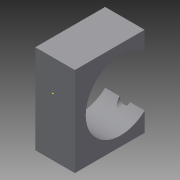
# Autodesk Inventor part: Noke_base
Saved by Autodesk Inventor 2015 SP2 (Build 190223200, 223)
## iProperties
Created: 2016-08-30
Part Number: Noke_base
Material: Generic
Document SubType Name: Modeling
Designer: jm799
Density: 1 g/cm^3
Appearance: Default
Author: jm799
Autodesk Inventor part; units mm, degrees
ref_plane "YZ Plane" through (0, 0, 0) normal (1, 0, 0) x (0, 1, 0)
ref_plane "XZ Plane" through (0, 0, 0) normal (0, 1, 0) x (-1, 0, 0)
ref_plane "XY Plane" through (0, 0, 0) normal (0, 0, 1) x (1, 0, 0)
sketch "Sketch1" plane through (0, 0, 0) normal (0, 1, 0) x (-1, 0, 0)
  line L0 (13.7338, 24.3615) -> (-17.2662, 24.3615)
  line L1 (-17.2662, 24.3615) -> (-17.2662, -45.6385)
  line L2 (-17.2662, -45.6385) -> (13.7338, -45.6385)
  line L3 (13.7338, -45.6385) -> (13.7338, 24.3615)
  point P0 (0, 0)
  dimension "d0" = 31
  dimension "d1" = 70
  constraints: 8 end point, 2 parallel, 1 horizontal, 1 perpendicular
  measures "d0" distance of L0.start L0.end
  measures "d1" distance of L0.end L1.end
extrude "Extrusion1" add sketch "Sketch1" along normal blind 54.75
sketch "Sketch2" plane through (17.2662, 0, 24.3615) normal (1, 0, 0) x (0, 0, -1)
  circle A0 centre (35, 35.9173) radius 27.375
  line L0 (0, 54.75) -> (70, 54.75) construction
  point P0 (24.3615, 0)
  point P1 (35, 54.75)
  dimension "d4" = 54.75
  constraints: 2 end point, 1 centre point, 1 horizontal, 1 midpoint, 1 vertical alignment
  measures "d4" diameter of A0
hole "Hole1" at (17.2662, 35.9173, -10.6385) direction (-1, 0, 0) diameter 54.75 end through all
sketch "Sketch3" plane through (0, 0, 0) normal (0, -1, 0) x (1, 0, 0)
  point P0 (0, 0)
sketch "Sketch4" plane through (0, 54.75, 0) normal (0, 1, 0) x (1, 0, 0)
  line L0 (-13.7338, -9.229) -> (17.2662, -9.229) construction
  line L1 (17.2662, -9.229) -> (-13.7338, -9.229) construction
  circle A0 centre (1.7662, -9.229) radius 4 construction
  point P0 (0, 0)
  dimension "d12" = 8
  constraints: 2 end point, 1 centre point, 1 horizontal, 1 midpoint
  measures "d12" diameter of A0
sketch "Sketch5" plane through (0, 54.75, 0) normal (0, 1, 0) x (1, 0, 0)
  line L0 (17.2662, 30.506) -> (-13.7338, 30.506) construction
  line L1 (-13.7338, 30.506) -> (17.2662, 30.506) construction
  circle A0 centre (1.7662, 30.506) radius 4 construction
  point P0 (0, 0)
  dimension "d13" = 8
  constraints: 2 end point, 1 centre point, 1 horizontal, 1 midpoint
  measures "d13" diameter of A0
hole "Hole2" at (1.7662, 54.75, 9.229) direction (0, -1, 0) diameter 8 depth 8 tip angle 118
hole "Hole3" at (1.7662, 54.75, -30.506) direction (0, -1, 0) diameter 8 depth 8 tip angle 118
sketch "Sketch6" plane through (0, 54.75, 0) normal (0, 1, 0) x (1, 0, 0)
  point P0 (0, 0)
body "Solid1"
